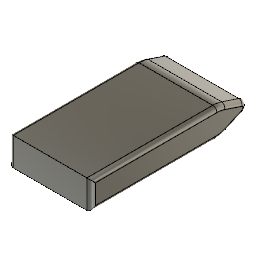
Monitor TFT v8 (Autodesk Fusion 360 archive; units mm, degrees)
design "LiPo 1200 10x28x53"
Autodesk Fusion 360 part; units mm, degrees
sketch "Skizze1" plane through (0, 0, 0) normal (1, 0, 0) x (0, 1, 0)
  line L0 (-10.6228, 0) -> (-55, 0)
  line L1 (-55, 0) -> (-55, -10)
  line L2 (-55, -10) -> (-11.1221, -10)
  line L3 (0, -4.7003) -> (0, -4.4415)
  line L4 (-7.4605, -0.5132) -> (-1.3675, -2.5442)
  line L5 (-7.0608, -9.1381) -> (-1.1877, -6.5279)
  arc A0 (-7.4605, -0.5132) -> (-10.6228, 0) centre (-10.6228, -10) ccw
  arc A1 (-11.1221, -10) -> (-7.0608, -9.1381) centre (-11.1221, 0) ccw
  arc A2 (0, -4.4415) -> (-1.3675, -2.5442) centre (-2, -4.4415) ccw
  arc A3 (-1.1877, -6.5279) -> (0, -4.7003) centre (-2, -4.7003) ccw
  dimension "d1" = 10
  dimension "d2" = 55
  dimension "d4" = 10
  dimension "d5" = 10
  dimension "d6" = 2
  dimension "d7" = 2
  constraint horizontal L0
  constraint vertical L1
  constraint horizontal L2
  constraint vertical L3
  constraint tangent L0 A0
  constraint tangent L4 A0
  constraint tangent L2 A1
  constraint tangent L5 A1
  constraint tangent L4 A2
  constraint tangent L3 A2
  constraint tangent L5 A3
  constraint tangent L3 A3
  measures "d1" distance of L0 L2
  measures "d2" distance of L1 L3
  measures "d4" radius of A0
  measures "d5" radius of A1
  measures "d6" radius of A2
  measures "d7" radius of A3
extrude "Extrusion1" add sketch "Skizze1" along normal blind 29
fillet "Abrundung1" radius 1.5 10 edges at (29, -33.0611, -10) (29, -9.0462, -9.7822) (29, -4.1242, -7.833) (29, -0.323, -5.7901) (29, 0, -4.5709) (29, -0.3775, -3.2721) (29, -4.414, -1.5287) (29, -9.021, -0.1291) (29, -32.8114, 0) (29, -55, -5)
fillet "Abrundung1" radius 1.5 10 edges at (0, -33.0611, -10) (0, -9.0462, -9.7822) (0, -4.1242, -7.833) (0, -0.323, -5.7901) (0, 0, -4.5709) (0, -0.3775, -3.2721) (0, -4.414, -1.5287) (0, -9.021, -0.1291) (0, -32.8114, 0) (0, -55, -5)
